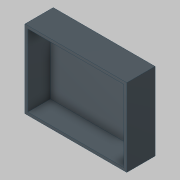
# Autodesk Inventor part: NA002
Saved by Autodesk Inventor 2017 (Build 210142000, 142)
## iProperties
Created: 2017-06-04
Part Number: NA002
Material: ABS Plastic
Document SubType Name: Modeling
Designer: Zach
Density: 1.06 g/cm^3
Appearance: CR Dark Blue
Author: Zach
Autodesk Inventor part; units mm, degrees
ref_plane "YZ Plane" through (0, 0, 0) normal (1, 0, 0) x (0, 1, 0)
ref_plane "XZ Plane" through (0, 0, 0) normal (0, 1, 0) x (-1, 0, 0)
ref_plane "XY Plane" through (0, 0, 0) normal (0, 0, 1) x (1, 0, 0)
sketch "Sketch1" plane through (0, 0, 0) normal (0, 0, 1) x (1, 0, 0)
  line L0 (0, 0) -> (180, 0)
  line L1 (180, 0) -> (180, -137.5)
  line L2 (180, -137.5) -> (0, -137.5)
  line L3 (0, -137.5) -> (0, 0)
  dimension "d0" = 180
  dimension "d1" = 137.5
  constraints: 8 end point, 2 parallel, 1 horizontal, 1 perpendicular
  measures "d0" distance of L1.end L2.end
  measures "d1" distance of L0.end L1.end
extrude "Extrusion1" add sketch "Sketch1" along normal blind 10
sketch "Sketch2" plane through (0, 0, 10) normal (0, 0, 1) x (1, 0, 0)
  circle A0 centre (35, -12.5) radius 2.5
  circle A1 centre (35, -37.5) radius 2.5
  line L0 (180, 0) -> (0, 0) projected
  line L1 (0, 0) -> (0, -137.5) projected
  circle A2 centre (145, -12.5) radius 2.5
  circle A3 centre (145, -37.5) radius 2.5
  line L2 (180, -137.5) -> (180, 0) projected
  dimension "d4" = 5
  dimension "d5" = 5
  dimension "d6" = 12.5
  dimension "d7" = 25
  dimension "d8" = 35
  dimension "d9" = 5
  dimension "d10" = 5
  dimension "d11" = 35
  constraints: 4 centre point, 2 horizontal alignment, 2 vertical alignment
  measures "d4" diameter of A0
  measures "d5" diameter of A1
  measures "d6" distance from line of A0.centre L0
  measures "d7" distance of A1.centre A0.centre
  measures "d8" distance from line of L1 A0.centre
  measures "d9" diameter of A2
  measures "d10" diameter of A3
  measures "d11" distance from line of L2 A2.centre
extrude "Extrusion2" cut sketch "Sketch2" against normal through all
sketch "Sketch3" plane through (0, 0, 10) normal (0, 0, 1) x (1, 0, 0)
  circle A0 centre (145, -12.5) radius 2.5 projected
  circle A1 centre (35, -12.5) radius 2.5 projected
  circle A2 centre (35, -37.5) radius 2.5 projected
  circle A3 centre (145, -37.5) radius 2.5 projected
  line L0 (180, 0) -> (0, 0) projected
  line L1 (0, 0) -> (0, -137.5) projected
  line L2 (0, -137.5) -> (180, -137.5) projected
  line L3 (180, -137.5) -> (180, 0) projected
  line L4 (5, -132.5) -> (5, -5)
  line L5 (5, -5) -> (175, -5)
  line L6 (175, -5) -> (175, -132.5)
  line L7 (175, -132.5) -> (5, -132.5)
  dimension "d14" = 5
  constraints: 8 end point, 3 other
  measures "d14" distance between parallel lines of L1 L4
extrude "Extrusion3" add sketch "Sketch3" along normal blind 40 contours L3 L2 L1 L0
sketch "Sketch4" plane through (0, 0, 10) normal (0, 0, 1) x (1, 0, 0)
  line L0 (175, -5) -> (5, -5) projected
  line L1 (80, -5) -> (100, -5)
  line L2 (100, -5) -> (100, -20)
  line L3 (100, -20) -> (80, -20)
  line L4 (80, -20) -> (80, -5)
  line L5 (0, 0) -> (0, -137.5) projected
  dimension "d17" = 20
  dimension "d18" = 15
  dimension "d19" = 80
  constraints: 8 end point, 2 parallel, 1 horizontal, 1 perpendicular, 1 point on line
  measures "d17" distance of L2.end L3.end
  measures "d18" distance of L1.end L2.end
  measures "d19" distance between parallel lines of L5 L4
extrude "Extrusion4" cut sketch "Sketch4" against normal through all
body "Solid1"
